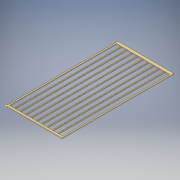
# Autodesk Inventor part: Lathhouse roof
Saved by Autodesk Inventor 2018 (Build 220112000, 112)
## iProperties
Created: 2019-05-09
Part Number: Lathhouse roof
Material: Generic
Document SubType Name: Modeling
Designer: 10043883
Density: 1 g/cm^3
Appearance: Wheat
Author: 10043883
Autodesk Inventor part; units mm, degrees
ref_plane "YZ Plane" through (0, 0, 0) normal (1, 0, 0) x (0, 1, 0)
ref_plane "XZ Plane" through (0, 0, 0) normal (0, 1, 0) x (-1, 0, 0)
ref_plane "XY Plane" through (0, 0, 0) normal (0, 0, 1) x (1, 0, 0)
sketch "Sketch1" plane through (0, 0, 0) normal (0, 1, 0) x (-1, 0, 0)
  line L0 (0, 0) -> (-18288, 0)
  line L1 (-18288, 0) -> (-18288, -36576)
  line L2 (-18288, -36576) -> (0, -36576)
  line L3 (0, -36576) -> (0, 0)
  dimension "d0" = 18288
  dimension "d1" = 36576
  constraints: 8 end point, 2 parallel, 1 horizontal, 1 perpendicular
  measures "d0" distance of L2.end L1.end
  measures "d1" distance of L1.end L0.end
extrude "Extrusion1" add sketch "Sketch1" along normal blind 254
sketch "Sketch2" plane through (0, 254, 0) normal (0, 1, 0) x (1, 0, 0)
  point P0 (0, 0)
sketch "Sketch4" plane through (0, 254, 0) normal (0, 1, 0) x (1, 0, 0)
  line L0 (417.1049, 605.6706) -> (417.1049, 35673.7899)
  line L1 (417.1049, 35673.7899) -> (1953.5948, 35673.7899)
  line L2 (1953.5948, 35673.7899) -> (1953.5948, 605.6706)
  line L3 (1953.5948, 605.6706) -> (417.1049, 605.6706)
  line L4 (3731.5948, 35673.7899) -> (3731.5948, 605.6706)
  line L5 (3731.5948, 605.6706) -> (2195.1049, 605.6706)
  line L6 (2195.1049, 605.6706) -> (2195.1049, 35673.7899)
  line L7 (2195.1049, 35673.7899) -> (3731.5948, 35673.7899)
  line L8 (5509.5948, 35673.7899) -> (5509.5948, 605.6706)
  line L9 (5509.5948, 605.6706) -> (3973.1049, 605.6706)
  line L10 (3973.1049, 605.6706) -> (3973.1049, 35673.7899)
  line L11 (3973.1049, 35673.7899) -> (5509.5948, 35673.7899)
  line L12 (7287.5948, 35673.7899) -> (7287.5948, 605.6706)
  line L13 (7287.5948, 605.6706) -> (5751.1049, 605.6706)
  line L14 (5751.1049, 605.6706) -> (5751.1049, 35673.7899)
  line L15 (5751.1049, 35673.7899) -> (7287.5948, 35673.7899)
  line L16 (9065.5948, 35673.7899) -> (9065.5948, 605.6706)
  line L17 (9065.5948, 605.6706) -> (7529.1049, 605.6706)
  line L18 (7529.1049, 605.6706) -> (7529.1049, 35673.7899)
  line L19 (7529.1049, 35673.7899) -> (9065.5948, 35673.7899)
  line L20 (10843.5948, 35673.7899) -> (10843.5948, 605.6706)
  line L21 (10843.5948, 605.6706) -> (9307.1049, 605.6706)
  line L22 (9307.1049, 605.6706) -> (9307.1049, 35673.7899)
  line L23 (9307.1049, 35673.7899) -> (10843.5948, 35673.7899)
  line L24 (12621.5948, 35673.7899) -> (12621.5948, 605.6706)
  line L25 (12621.5948, 605.6706) -> (11085.1049, 605.6706)
  line L26 (11085.1049, 605.6706) -> (11085.1049, 35673.7899)
  line L27 (11085.1049, 35673.7899) -> (12621.5948, 35673.7899)
  line L28 (14399.5948, 35673.7899) -> (14399.5948, 605.6706)
  line L29 (14399.5948, 605.6706) -> (12863.1049, 605.6706)
  line L30 (12863.1049, 605.6706) -> (12863.1049, 35673.7899)
  line L31 (12863.1049, 35673.7899) -> (14399.5948, 35673.7899)
  line L32 (16177.5948, 35673.7899) -> (16177.5948, 605.6706)
  line L33 (16177.5948, 605.6706) -> (14641.1049, 605.6706)
  line L34 (14641.1049, 605.6706) -> (14641.1049, 35673.7899)
  line L35 (14641.1049, 35673.7899) -> (16177.5948, 35673.7899)
  line L36 (17955.5948, 35673.7899) -> (17955.5948, 605.6706)
  line L37 (17955.5948, 605.6706) -> (16419.1049, 605.6706)
  line L38 (16419.1049, 605.6706) -> (16419.1049, 35673.7899)
  line L39 (16419.1049, 35673.7899) -> (17955.5948, 35673.7899)
  point P0 (0, 0)
  dimension "d15" = 1778
  constraints: 80 end point, 3 perpendicular, 1 collinear, 1 horizontal, 1 vertical, 71 other
  measures "d15" distance of L1.end L4.start
extrude "Extrusion3" cut sketch "Sketch4" against normal through all
body "Solid1"
